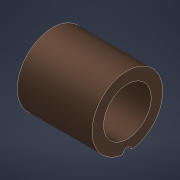
# Autodesk Inventor part: Втулка
Saved by Autodesk Inventor 2021 (Build 250183000, 183)
## iProperties
Created: 2022-05-01
Part Number: Втулка
Material: Bronze, Cast
Document SubType Name: Modeling
Designer: DuctopwH
Density: 8.87 g/cm^3
Appearance: Bronze - Satin
Author: DuctopwH
Autodesk Inventor part; units mm, degrees
ref_plane "YZ Plane" through (0, 0, 0) normal (1, 0, 0) x (0, 1, 0)
ref_plane "XZ Plane" through (0, 0, 0) normal (0, 1, 0) x (-1, 0, 0)
ref_plane "XY Plane" through (0, 0, 0) normal (0, 0, 1) x (1, 0, 0)
sketch "Sketch1" plane through (0, 0, 0) normal (0, 0, 1) x (1, 0, 0)
  line L0 (0, 0) -> (-55, 0)
  line L1 (-55, 26) -> (0, 26)
  line L2 (0, 26) -> (0, 17.5)
  line L3 (0, 17.5) -> (-55, 17.5)
  line L4 (-55, 17.5) -> (-55, 26)
  dimension "d0" = 35
  dimension "d1" = 52
  dimension "d2" = 55
  constraints: 10 end point, 2 horizontal, 2 parallel, 2 point on line, 1 perpendicular
  measures "d0" diameter of L3 L0
  measures "d1" diameter of L1 L0
  measures "d2" distance between parallel lines of L2 L4
revolve "Revolution1" add sketch "Sketch1" angle 360 about axis through (0, 0, 0) along (-1, 0, 0)
sketch "Sketch2" plane through (0, 0, 0) normal (1, 0, 0) x (0, 0, -1)
  line L0 (0, 0) -> (0, -26)
  circle A0 centre (0, 0) radius 26 projected
  constraints: 2 end point, 1 coincident, 1 vertical, 1 vertical alignment, 1 other
hole "Hole1" at (0, -26, 0) direction (-1, 0, 0) diameter 6.917 depth 25 thread size "M8x1" class "6H" standard "ANSI Metric M Profile"
body "Solid1"
